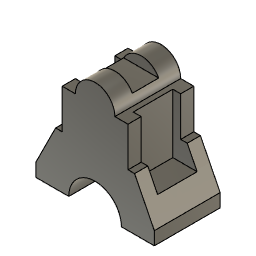
Sketch12_Final v0 (Autodesk Fusion 360 design; units mm, degrees)
Autodesk Fusion 360 part; units mm, degrees
sketch "Sketch1" plane through (0, 0, 0) normal (0, 1, 0) x (1, 0, 0)
  line L0 (-20, 0) -> (-45, 0)
  line L1 (-45, 0) -> (-45, -10)
  line L2 (45, 0) -> (45, -10)
  arc A0 (-20, 0) -> (20, 0) centre (0, 0) ccw
  line L3 (20, 0) -> (45, 0)
  line L4 (0, 0) -> (0, -40)
  line L5 (25, -40) -> (30, -40)
  line L6 (-25, -40) -> (-30, -40)
  line L7 (-30, -40) -> (-45, -10)
  line L8 (30, -40) -> (45, -10)
  line L9 (-25, -40) -> (-25, -70)
  line L10 (25, -40) -> (25, -70)
  arc A1 (-15, -70) -> (15, -70) centre (0, -70) ccw
  line L11 (-25, -70) -> (-15, -70)
  line L12 (15, -70) -> (25, -70)
  dimension "d1" = 45
  dimension "d2" = 45
  dimension "d3" = 40
  dimension "d4" = 10
  dimension "d5" = 10
  dimension "d6" = 40
  dimension "d7" = 30
  dimension "d8" = 30
  dimension "d9" = 25
  dimension "d10" = 25
  dimension "d11" = 30
  dimension "d12" = 30
  dimension "d13" = 30
  constraint coincident A0.centre L4.start
  constraint perpendicular L0 L1
  constraint perpendicular L2 L3
  constraint perpendicular L3 L4
  constraint perpendicular L4 L5
  constraint perpendicular L4 L6
  constraint coincident A1.end L11
  constraint collinear L11 L12
  constraint coincident A1.centre L11
  measures "d1" distance of A0.centre L2.start
  measures "d2" distance of A0.centre L0.end
  measures "d3" diameter of A0
  measures "d4" distance of L0.end L1.end
  measures "d5" distance of L2.start L2.end
  measures "d6" distance of A0.centre L4.end
  measures "d7" distance of L4.end L5.end
  measures "d8" distance of L4.end L6.end
  measures "d9" distance of L4.end L6.start
  measures "d10" distance of L4.end L5.start
  measures "d11" distance of L6.start L9.end
  measures "d12" distance of L5.start L10.end
  measures "d13" diameter of A1
extrude "Extrude1" add sketch "Sketch1" along normal mid plane 50
sketch "Sketch2" plane through (-45, 0, 0) normal (-1, 0, 0) x (0, -1, 0)
  line L0 (25, 10) -> (-25, 10)
  line L1 (-25, 10) -> (-25, 0)
  line L2 (-25, 0) -> (25, 0)
  line L3 (25, 0) -> (25, 10)
  line L4 (-15, 70) -> (15, 70)
  line L5 (15, 70) -> (15, 40)
  line L6 (-15, 70) -> (-15, 25)
  line L7 (15, 70) -> (15, 25)
  line L8 (15, 25) -> (-15, 25)
  dimension "d17" = 30
  dimension "d19" = 30
  dimension "d20" = 45
  dimension "d21" = 45
  constraint perpendicular L4 L5
  constraint perpendicular L4 L6
  constraint perpendicular L4 L7
  measures "d17" distance of L4.start L4.end
  measures "d19" distance of L4.end L5.end
  measures "d20" distance of L4.start L6.end
  measures "d21" distance of L4.end L7.end
extrude "Extrude2" cut sketch "Sketch2" along normal blind 30 from surface at -26 contours L4 L5 L6 L7 L8
sketch "Sketch4" plane through (0, 0, 0) normal (1, 0, 0) x (0, 1, 0)
  line L0 (-15, 70) -> (15, 70)
  line L1 (15, 70) -> (15, 25)
  line L2 (-15, 70) -> (-15, 25)
  line L3 (-15, 25) -> (15, 25)
  dimension "d30" = 30
  dimension "d31" = 45
  dimension "d32" = 45
  dimension "d33" = 30
  constraint perpendicular L0 L1
  constraint perpendicular L0 L2
  constraint perpendicular L2 L3
  measures "d30" distance of L0.start L0.end
  measures "d31" distance of L0.end L1.end
  measures "d32" distance of L0.start L2.end
  measures "d33" distance of L2.end L1.end
extrude "Extrude3" cut sketch "Sketch4" along normal blind 20 from surface at 19
sketch "Sketch5" plane through (0, 0, 0) normal (0, 0, 1) x (1, 0, 0)
  line L0 (-15, -10) -> (-15, 10)
  line L1 (-15, 10) -> (15, 10)
  line L2 (15, 10) -> (15, -10)
  line L3 (15, -10) -> (-15, -10)
  dimension "d38" = 20
  dimension "d40" = 20
  constraint perpendicular L1 L2
  measures "d38" distance of L0.start L0.end
  measures "d40" distance of L1.end L2.end
extrude "Extrude4" cut sketch "Sketch5" along normal blind 10 from surface at 77
